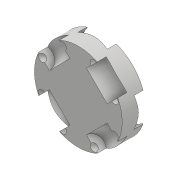
# Autodesk Inventor part: wheel_core_template
Saved by Autodesk Inventor 2017 (Build 210142000, 142)
## iProperties
Created: 2018-10-27
Part Number: wheel_core_template
Material: Generic
Document SubType Name: Modeling
Designer: mfans
Density: 1 g/cm^3
Appearance: Default
Author: mfans
Autodesk Inventor part; units mm, degrees
ref_plane "YZ Plane" through (0, 0, 0) normal (1, 0, 0) x (0, 1, 0)
ref_plane "XZ Plane" through (0, 0, 0) normal (0, 1, 0) x (-1, 0, 0)
ref_plane "XY Plane" through (0, 0, 0) normal (0, 0, 1) x (1, 0, 0)
sketch "Sketch1" plane through (0, 0, 0) normal (0, 1, 0) x (-1, 0, 0)
  circle A0 centre (0, 0) radius 30
  dimension "d0" = 60
  constraints: 1 centre point, 1 coincident
  measures "d0" diameter of A0
extrude "Extrusion1" add sketch "Sketch1" along normal mid plane 16
sketch "Sketch2" plane through (0, 8, 0) normal (0, 1, 0) x (1, 0, 0)
  line L0 (18, 10) -> (18, -10)
  line L1 (18, -10) -> (25, -10)
  line L2 (32, -10) -> (32, 10)
  line L3 (32, 10) -> (18, -10) construction
  line L4 (18, 10) -> (32, -10) construction
  line L5 (25, 0) -> (31, 0)
  arc A0 (25, -7.5) -> (25, -12.5) centre (25, -10) ccw
  arc A1 (25, 12.5) -> (25, 7.5) centre (25, 10) ccw
  line L6 (25, -12.5) -> (25, 12.5)
  line L7 (32, 10) -> (27.5, 10)
  line L8 (25, 10) -> (18, 10)
  point P0 (0, 0)
  dimension "d3" = 14
  dimension "d4" = 25
  dimension "d5" = 6
  dimension "d6" = 5
  dimension "d7" = 5
  dimension "d8" = 20
  constraints: 18 end point, 4 point on circle, 4 point on line, 3 horizontal, 3 parallel, 2 centre point, 2 midpoint, 2 perpendicular, 1 vertical
  measures "d3" distance of L2.end L0.start
  measures "d4" distance of point (0, 0) L5.start
  measures "d5" distance of L5.start L5.end
  measures "d6" diameter of A0
  measures "d7" diameter of A1
  measures "d8" distance of L0.start L0.end
sketch "Sketch2 outline for Revolution1" plane through (0, 8, 0) normal (0, 1, 0) x (1, 0, 0)
  arc A0 (25, 12.5) -> (22.5, 10) centre (25, 10) ccw
  line L0 (22.5, 10) -> (18, 10)
  line L1 (18, 10) -> (18, -10)
  line L2 (18, -10) -> (22.5, -10)
  arc A1 (22.5, -10) -> (25, -12.5) centre (25, -10) ccw
  line L3 (25, -12.5) -> (25, 12.5)
revolve "Revolution1" cut sketch "Sketch2 outline for Revolution1" angle 360 about axis through (25, 8, 12.5) along (0, 0, -1)
pattern_circular "Circular Pattern2" count 4 over 360 about axis through (0, -10, 0) along (0, 1, 0) of "Revolution1"
sketch "Sketch3" plane through (0, -8, 0) normal (0, -1, 0) x (1, 0, 0)
  line L0 (0, 0) -> (0, 30)
  circle A0 centre (0, 0) radius 30
  line L1 (19.79899, 5.656854) -> (5.656854, 19.79899)
  line L2 (15.556349, 29.698485) -> (29.698485, 15.556349)
  line L3 (19.79899, 5.656854) -> (15.556349, 29.698485) construction
  line L4 (5.656854, 19.79899) -> (29.698485, 15.556349) construction
  line L5 (0, 0) -> (17.67767, 17.67767)
  line L6 (21.213203, 21.213203) -> (21.429204, 21.429204)
  arc A1 (22.98097, 12.374369) -> (26.516504, 8.838835) centre (24.748737, 10.606602) ccw
  arc A2 (8.838835, 26.516504) -> (12.374369, 22.98097) centre (10.606602, 24.748737) ccw
  line L7 (26.516504, 8.838835) -> (8.838835, 26.516504)
  line L8 (29.698485, 15.556349) -> (27.071068, 12.928932)
  line L9 (24.748737, 10.606602) -> (19.79899, 5.656854)
  line L10 (5.656854, 19.79899) -> (10.606602, 24.748737)
  line L11 (12.374369, 26.516504) -> (15.556349, 29.698485)
  dimension "d17" = 25
  dimension "d18" = 14
  dimension "d19" = 20
  dimension "d20" = 5
  dimension "d21" = 5
  constraints: 24 end point, 7 point on circle, 5 parallel, 4 perpendicular, 4 point on line, 2 centre point, 2 midpoint, 1 vertical
  measures "d17" distance of L0.start L5.end
  measures "d18" distance of L1.end L2.start
  measures "d19" distance of L1.start L1.end
  measures "d20" diameter of A1
  measures "d21" diameter of A2
sketch "Sketch3 outline for Revolution2" plane through (0, -8, 0) normal (0, -1, 0) x (1, 0, 0)
  arc A0 (8.838835, 26.516504) -> (8.838835, 22.98097) centre (10.606602, 24.748737) ccw
  line L0 (8.838835, 22.98097) -> (5.656854, 19.79899)
  line L1 (5.656854, 19.79899) -> (19.79899, 5.656854)
  line L2 (19.79899, 5.656854) -> (22.98097, 8.838835)
  arc A1 (22.98097, 8.838835) -> (26.516504, 8.838835) centre (24.748737, 10.606602) ccw
  line L3 (26.516504, 8.838835) -> (8.838835, 26.516504)
revolve "Revolution2" cut sketch "Sketch3 outline for Revolution2" angle 360 about axis through (26.516504, -8, 8.838835) along (-0.7071068, 0, 0.7071068)
pattern_circular "Circular Pattern3" count 4 over 360 about axis through (0, -10, 0) along (0, 1, 0) of "Revolution2"
body "Solid1"
